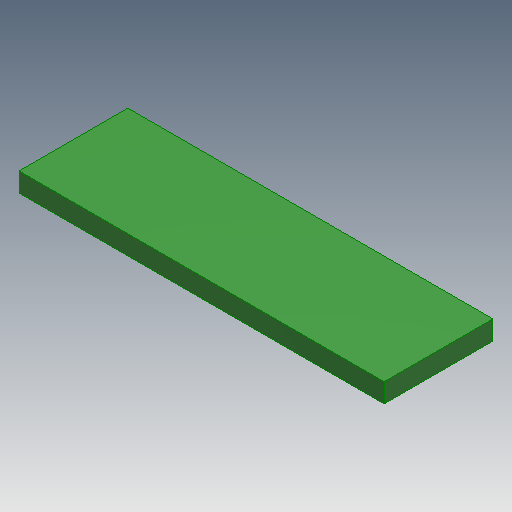
# Autodesk Inventor part: LOGO-SFENEW
Saved by Autodesk Inventor 2017 (Build 210142000, 142)
## iProperties
Part Number: LOGO-SFENEW
Material: Generisch
Document SubType Name: Modeling
Designer: Werkstatt
Density: 1 g/cm^3
Appearance: SFE-NEW-WEBLOGO, LOGO-SFENEW
Author: Werkstatt
Autodesk Inventor part; units mm, degrees
ref_plane "YZ Plane" through (0, 0, 0) normal (1, 0, 0) x (0, 1, 0)
ref_plane "XZ Plane" through (0, 0, 0) normal (0, 1, 0) x (-1, 0, 0)
ref_plane "XY Plane" through (0, 0, 0) normal (0, 0, 1) x (1, 0, 0)
sketch "SFE-NEW-WEBLOGO, LOGO-SFENEW_60" plane through (0, 0, 0) normal (0, 0, 1) x (1, 0, 0)
  line L0 (0.0127, 5.6871) -> (19.0373, 5.6871)
  line L1 (19.0373, 5.6871) -> (19.0373, 0.0178)
  line L2 (19.0373, 0.0178) -> (0.0127, 0.0178)
  line L3 (0.0127, 0.0178) -> (0.0127, 5.6871)
  constraints: 8 end point
extrude "Extrusion1" add sketch "SFE-NEW-WEBLOGO, LOGO-SFENEW_60" along normal blind 1
